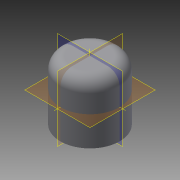
# Autodesk Inventor part: Sirene
Saved by Autodesk Inventor 2015 (Build 190159000, 159)
## iProperties
Created: 2019-02-16
Part Number: Sirene
Material: Generisch
Document SubType Name: Modeling
Designer: Boris
Density: 1 g/cm^3
Appearance: Vorgabe
Author: Boris
Autodesk Inventor part; units mm, degrees
sketch "Skizze1" plane through (0, 0, 0) normal (0, 0, 1) x (1, 0, 0)
  circle A0 centre (0, 0) radius 5
  line L0 (0, 81.3997) -> (0, -19.4) projected
  circle A1 centre (0, 0) radius 4.25
  point P0 (37.012, 66.9998)
  dimension "d0" = 10
  dimension "d1" = 8.5
  constraints: 2 centre point, 1 coincident
  measures "d0" diameter of A0
  measures "d1" diameter of A1
extrude "Extrusion1" add sketch "Skizze1" along normal mid plane 10 contours A0 L0 A1 | L0 A1 A0
sketch "Skizze2" plane through (0, 0, 5) normal (0, 0, 1) x (1, 0, 0)
  circle A0 centre (0, 0) radius 5 projected
extrude "Extrusion2" add sketch "Skizze2" against normal blind 2
fillet "Rundung1" radius 2 1 edges at (-4.25, 0, 3)
fillet "Rundung2" radius 2 1 edges at (-5, 0, 5)
